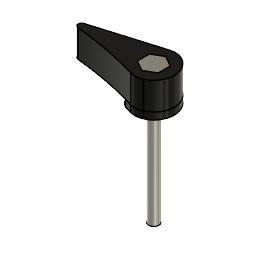
LB6 - 15° Tripod Leveling Attachment with ⅜” Mounting Screw (Autodesk Fusion 360 archive; units mm, degrees)
design "Lever (LB6)"
Autodesk Fusion 360 part; units mm, degrees
sketch "Sketch1" plane through (0, 0, 0) normal (0, 0, 1) x (1, 0, 0)
  circle A0 centre (0, 0) radius 1.5
  dimension "d1" = 3
  constraint coincident A0.centre origin
  measures "d1" diameter of A0
extrude "Extrude1" add sketch "Sketch1" along normal blind 28 makes body 1
sketch "Sketch2" plane through (0, 0, 28) normal (0, 0, 1) x (-1, 0, 0)
  circle A0 centre (0, 0) radius 1.5
  circle A1 centre (0, 0) radius 3
  dimension "d4" = 6
  constraint coincident A0.centre A1.centre
  measures "d4" diameter of A1
extrude "Extrude2" add sketch "Sketch2" along normal blind 2 contours A0 | A1 bodies 1
sketch "Sketch3" plane through (0, 0, 30) normal (0, 0, 1) x (-1, 0, 0)
  circle A0 centre (0, 0) radius 3
  line L0 (0, -3.5) -> (3.0311, -1.75)
  line L1 (3.0311, -1.75) -> (3.0311, 1.75)
  line L2 (3.0311, 1.75) -> (0, 3.5)
  line L3 (0, 3.5) -> (-3.0311, 1.75)
  line L4 (-3.0311, 1.75) -> (-3.0311, -1.75)
  line L5 (-3.0311, -1.75) -> (0, -3.5)
  dimension "d7" = 3.5
  constraint coincident A0.centre origin
  constraint vertical L4
  measures "d7" distance of L0.start A0.centre
extrude "Extrude3" add sketch "Sketch3" along normal blind 10 contours A0 | L0 L1 L2 L3 L4 L5 bodies 1
sketch "Sketch4" plane through (0, 0, 40) normal (0, 0, 1) x (-1, 0, 0)
  line L0 (-3.0311, -1.75) -> (0, -3.5)
  line L1 (0, -3.5) -> (3.0311, -1.75)
  line L2 (3.0311, -1.75) -> (3.0311, 1.75)
  line L3 (3.0311, 1.75) -> (0, 3.5)
  line L4 (0, 3.5) -> (-3.0311, 1.75)
  line L5 (-3.0311, 1.75) -> (-3.0311, -1.75)
  line L6 (1.0405, -5.7108) -> (20.2864, 0.0419)
  arc A0 (0.9798, 5.7098) -> (20.1005, 1.9949) centre (30.843, 108.3515) ccw
  arc A1 (20.2864, 0.0419) -> (20.1005, 1.9949) centre (20, 1) ccw
  arc A2 (-2.502, 5.4535) -> (-2.3485, -5.5213) centre (0, 0) ccw
  arc A3 (-2.3485, -5.5213) -> (1.0405, -5.7108) centre (-0.3914, -0.9202) ccw
  arc A4 (0.9798, 5.7098) -> (-2.502, 5.4535) centre (-0.417, 0.9089) ccw
  dimension "d10" = 12
  dimension "d12" = 1
  dimension "d13" = 20
  dimension "d14" = 5
  dimension "d20" = 5
  dimension "d21" = 106.8978
  dimension "d22" = 0.8298
  dimension "d23" = 2.6141
  dimension "d24" = 33.8741
  constraint coincident A2.centre origin
  constraint tangent L6 A1
  constraint tangent A0 A1
  constraint tangent L6 A3
  constraint tangent A2 A3
  constraint tangent A0 A4
  constraint tangent A2 A4
  measures "d10" diameter of A2
  measures "d12" radius of A1
  measures "d13" horizontal distance of A2.centre A1.centre
  measures "d14" radius of A3
  measures "d20" radius of A4
  measures "d21" radius of A0
  measures "d22" vertical distance of L0.start A3.centre
  measures "d23" distance of L5 A4.centre
  measures "d24" distance of L5 A0.centre
extrude "Extrude4" add sketch "Sketch4" against normal blind 8 separate body makes body 2
sketch "Sketch5" plane through (0, 0, 32) normal (0, 0, -1) x (1, 0, 0)
  line L0 (3.0311, 1.75) -> (3.0311, -1.75)
  line L1 (3.0311, -1.75) -> (0, -3.5)
  line L2 (0, -3.5) -> (-3.0311, -1.75)
  line L3 (-3.0311, -1.75) -> (-3.0311, 1.75)
  line L4 (-3.0311, 1.75) -> (0, 3.5)
  line L5 (0, 3.5) -> (3.0311, 1.75)
  arc A0 (2.3485, -5.5213) -> (2.502, 5.4535) centre (0, 0) ccw
  arc A1 (-20.1005, 1.9949) -> (-0.9798, 5.7098) centre (-30.843, 108.3515) ccw
  arc A2 (-20.1005, 1.9949) -> (-20.2864, 0.0419) centre (-20, 1) ccw
  line L6 (-20.2864, 0.0419) -> (-1.0405, -5.7108)
  arc A3 (-1.0405, -5.7108) -> (2.3485, -5.5213) centre (0.3914, -0.9202) ccw
  circle A4 centre (0, 0) radius 6
  arc A5 (2.502, 5.4535) -> (-0.9798, 5.7098) centre (0.417, 0.9089) ccw
  dimension "d17" = 12
  constraint coincident A0.centre A4.centre
  measures "d17" diameter of A4
extrude "Extrude5" add sketch "Sketch5" along normal blind 2 separate body contours A0 A1 L6 A3 A4 A5 makes body 3
equation "d2 = ( 55 / 2 ) * 1 mm + 0.5 mm"
